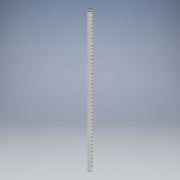
# Autodesk Inventor part: Ground_Antenna230mm_Support
Saved by Autodesk Inventor 2018 (Build 220112000, 112)
## iProperties
Created: 2018-10-12
Part Number: Ground_Antenna230mm_Support
Material: PVC-Piping
Document SubType Name: Modeling
Designer: Bradley
Density: 1.4 g/cm^3
Appearance: Smooth - White
Mass: 617.957 g
Surface Area: 2284.9 cm^2
Volume: 441.398 cm^3
Author: Bradley
Autodesk Inventor part; units mm, degrees
ref_plane "YZ Plane" through (0, 0, 0) normal (1, 0, 0) x (0, 1, 0)
ref_plane "XZ Plane" through (0, 0, 0) normal (0, 1, 0) x (-1, 0, 0)
ref_plane "XY Plane" through (0, 0, 0) normal (0, 0, 1) x (1, 0, 0)
sketch "Sketch1" plane through (0, 0, 0) normal (0, 0, 1) x (1, 0, 0)
  circle A0 centre (0, 0) radius 16.7005
  circle A1 centre (0, 0) radius 12.7
  dimension "d0" = 33.401
  dimension "d1" = 25.4
  constraints: 2 centre point, 2 coincident
  measures "d0" diameter of A0
  measures "d1" diameter of A1
extrude "Extrusion1" add sketch "Sketch1" along normal mid plane 1225
sketch "Sketch2" plane through (0, 0, 0) normal (1, 0, 0) x (0, 1, 0)
  line L0 (12.7, -612.5) -> (-12.7, -612.5) projected
  line L1 (12.7, -612.5) -> (-12.7, -612.5) projected
  line L2 (-12.7, 612.5) -> (12.7, 612.5) projected
  line L3 (-16.7005, -612.5) -> (-16.7005, 612.5) projected
  point P0 (0, 0)
  point P1 (0, -572.4235)
  point P2 (0, -612.5)
  point P3 (0, -545.2735)
  point P4 (0, -518.1235)
  point P5 (0, -490.9735)
  point P6 (0, -463.8235)
  point P7 (0, -436.6735)
  point P8 (0, -409.5235)
  point P9 (0, -382.3735)
  point P10 (0, -355.2235)
  point P11 (0, -328.0735)
  point P12 (0, -300.9235)
  point P13 (0, -273.7735)
  point P14 (0, -246.6235)
  point P15 (0, -219.4735)
  point P16 (0, -192.3235)
  point P17 (0, -165.1735)
  point P18 (0, -138.0235)
  point P19 (0, -110.8735)
  point P20 (0, -83.7235)
  point P21 (0, -56.5735)
  point P22 (0, -29.4235)
  point P23 (0, -2.2735)
  point P24 (0, 24.8765)
  point P25 (0, 52.0265)
  point P26 (0, 79.1765)
  point P27 (0, 106.3265)
  point P28 (0, 133.4765)
  point P29 (0, 160.6265)
  point P30 (0, 187.7765)
  point P31 (0, 214.9265)
  point P32 (0, 242.0765)
  point P33 (0, 269.2265)
  point P34 (0, 296.3765)
  point P35 (0, 323.5265)
  point P36 (0, 350.6765)
  point P37 (0, 377.8265)
  point P38 (0, 404.9765)
  point P39 (0, 432.1265)
  point P40 (0, 459.2765)
  point P41 (0, 486.4265)
  point P42 (0, 513.5765)
  point P43 (0, 540.7265)
  point P44 (0, 567.8765)
  point P45 (0, 595.0265)
  dimension "d4" = 40.0765
  dimension "d7" = 27.15
  constraints: 1 midpoint, 1 vertical, 1 vertical alignment, 43 other
  measures "d4" distance from line of L0 point (0, -572.423)
  measures "d7" distance of point (0, -572.423) point (0, -545.274)
hole "Hole1" at (0, 0, -572.4235) at (0, 0, -545.2735) at (0, 0, -518.1235) at (0, 0, -490.9735) at (0, 0, -463.8235) at (0, 0, -436.6735) at (0, 0, -409.5235) at (0, 0, -382.3735) at (0, 0, -355.2235) at (0, 0, -328.0735) at (0, 0, -300.9235) at (0, 0, -273.7735) at (0, 0, -246.6235) at (0, 0, -219.4735) at (0, 0, -192.3235) at (0, 0, -165.1735) at (0, 0, -138.0235) at (0, 0, -110.8735) at (0, 0, -83.7235) at (0, 0, -56.5735) at (0, 0, -29.4235) at (0, 0, -2.2735) at (0, 0, 24.8765) at (0, 0, 52.0265) at (0, 0, 79.1765) at (0, 0, 106.3265) at (0, 0, 133.4765) at (0, 0, 160.6265) at (0, 0, 187.7765) at (0, 0, 214.9265) at (0, 0, 242.0765) at (0, 0, 269.2265) at (0, 0, 296.3765) at (0, 0, 323.5265) at (0, 0, 350.6765) at (0, 0, 377.8265) at (0, 0, 404.9765) at (0, 0, 432.1265) at (0, 0, 459.2765) at (0, 0, 486.4265) at (0, 0, 513.5765) at (0, 0, 540.7265) at (0, 0, 567.8765) at (0, 0, 595.0265) direction (-1, 0, 0) diameter 6.35 end through all both
body "Solid1"
